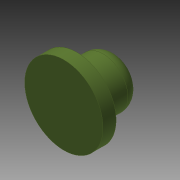
# Autodesk Inventor part: btn
Saved by Autodesk Inventor 2014 (Build 180170000, 170)
## iProperties
Created: 2017-11-14
Part Number: btn
Material: Типовые
Document SubType Name: Modeling
Designer: Nikopol
Density: 1 g/cm^3
Appearance: Оливково-зеленый
Author: Nikopol
Autodesk Inventor part; units mm, degrees
ref_plane "YZ Plane" through (0, 0, 0) normal (1, 0, 0) x (0, 1, 0)
ref_plane "XZ Plane" through (0, 0, 0) normal (0, 1, 0) x (-1, 0, 0)
ref_plane "XY Plane" through (0, 0, 0) normal (0, 0, 1) x (1, 0, 0)
sketch "Эскиз1" plane through (0, 0, 0) normal (0, 1, 0) x (-1, 0, 0)
  circle A0 centre (0, 0) radius 3
  dimension "d0" = 6
  constraints: 1 centre point, 1 coincident
  measures "d0" diameter of A0
extrude "Выдавливание1" add sketch "Эскиз1" along normal blind 1
sketch "Эскиз2" plane through (0, 1, 0) normal (0, 1, 0) x (1, 0, 0)
  circle A0 centre (0, 0) radius 3 projected
  circle A1 centre (0, 0) radius 1.9
  dimension "d3" = 3.8
  constraints: 1 centre point, 1 coincident
  measures "d3" diameter of A1
extrude "Выдавливание2" add sketch "Эскиз2" along normal blind 3 contours A1
fillet "Сопряжение1" radius 1 1 edges at (-1.9, 4, 0)
